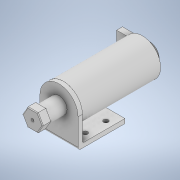
# Autodesk Inventor part: motor
Saved by Autodesk Inventor 2022 (Build 260153000, 153)
## iProperties
Created: 2022-07-16
Part Number: motor
Material: Типовые
Document SubType Name: Modeling
Designer: akapu
Density: 1 g/cm^3
Appearance: По умолчанию
Author: akapu
Autodesk Inventor part; units mm, degrees
ref_plane "YZ Plane" through (0, 0, 0) normal (1, 0, 0) x (0, 1, 0)
ref_plane "XZ Plane" through (0, 0, 0) normal (0, 1, 0) x (-1, 0, 0)
ref_plane "XY Plane" through (0, 0, 0) normal (0, 0, 1) x (1, 0, 0)
sketch "Эскиз1" plane through (0, 0, 0) normal (0, 1, 0) x (-1, 0, 0)
  line L0 (0, 0) -> (-26, 0)
  line L1 (0, -32) -> (-26, -32)
  line L2 (-26, -32) -> (0, -32)
  line L3 (0, -32) -> (0, 0)
  line L4 (0, 0) -> (-26, 0)
  line L5 (-26, 0) -> (-26, -32)
  constraints: 12 end point, 2 horizontal, 2 parallel, 1 perpendicular
extrude "Выдавливание1" add sketch "Эскиз1" along normal blind 3
sketch "Эскиз2" plane through (0, 3, 0) normal (0, 1, 0) x (1, 0, 0)
  line L0 (0, 0) -> (26, 0) projected
  line L1 (26, 0) -> (26, 33) projected
  line L2 (0, 0) -> (26, 0)
  line L3 (26, 0) -> (26, 3)
  line L4 (26, 3) -> (0, 3)
  line L5 (0, 3) -> (0, 0)
  dimension "d4" = 3
  constraints: 8 end point, 2 parallel, 1 horizontal, 1 perpendicular, 1 point on line
  measures "d4" distance of L3.end L2.end
extrude "Выдавливание2" add sketch "Эскиз2" along normal blind 30
sketch "Эскиз3" plane through (26, 3, -3) normal (0, 0, -1) x (-1, 0, 0)
  line L0 (0, 0) -> (26, 0) projected
  line L1 (13, 0) -> (13, 5)
  line L2 (13, 5) -> (13, 17.5)
  circle A0 centre (13, 17.5) radius 12.5
  point P0 (26, -3)
  dimension "d7" = 5
  dimension "d8" = 12.5
  constraints: 4 end point, 1 coincident, 1 midpoint, 1 point on line, 1 vertical, 1 vertical alignment, 2 other
  measures "d7" distance of L1.start L1.end
  measures "d8" distance of L1.end L2.end
extrude "Выдавливание3" add sketch "Эскиз3" along normal blind 61.8
sketch "Эскиз4" plane through (13, 20.5, -64.8) normal (0, 0, -1) x (-1, 0, 0)
  circle A0 centre (0, 0) radius 6.5
  circle A1 centre (0, 0) radius 12.5
  point P0 (13, -20.5)
  dimension "d11" = 13
  constraints: 2 centre point, 1 coincident
  measures "d11" diameter of A0
extrude "Выдавливание4" cut sketch "Эскиз4" against normal blind 8
sketch "Эскиз5" plane through (13, 20.5, -64.8) normal (0, 0, -1) x (-1, 0, 0)
  circle A0 centre (0, 0) radius 1
  circle A1 centre (0, 0) radius 6.5
  point P0 (13, -20.5)
  dimension "d14" = 2
  constraints: 2 centre point, 1 coincident
  measures "d14" diameter of A0
extrude "Выдавливание5" cut sketch "Эскиз5" against normal blind 3
sketch "Эскиз6" plane through (13, 20.5, -56.8) normal (0, 0, -1) x (-1, 0, 0)
  circle A0 centre (0, 0) radius 12.5 projected
  line L0 (-12.5, 0) -> (8.5, 0)
  line L1 (8.5, 0) -> (8.5, 7)
  line L2 (8.5, 7) -> (17.5, 7)
  line L3 (17.5, 7) -> (17.5, -7)
  line L4 (17.5, -7) -> (8.5, -7)
  line L5 (8.5, -7) -> (8.5, 0)
  point P0 (13, -20.5)
  dimension "d17" = 21
  dimension "d18" = 7
  dimension "d19" = 9
  dimension "d20" = 14
  constraints: 12 end point, 5 perpendicular, 1 horizontal, 1 horizontal alignment, 1 point on line, 1 other
  measures "d17" distance of L0.start L0.end
  measures "d18" distance of L0.end L1.end
  measures "d19" distance of L1.end L2.end
  measures "d20" distance of L2.end L3.end
extrude "Выдавливание6" add sketch "Эскиз6" along normal blind 4 contours A0 L4 L5 L1 L2 | A0 L2 L3 L4
sketch "Эскиз7" plane through (0, 0, 0) normal (0, 0, 1) x (1, 0, 0)
  circle A0 centre (13, 20.5) radius 1 projected
  circle A1 centre (13, 20.5) radius 5.5
  point P0 (0, 0)
  dimension "d23" = 11
  constraints: 1 centre point, 1 coincident
  measures "d23" diameter of A1
extrude "Выдавливание7" add sketch "Эскиз7" along normal blind 12 contours A0 | A1
sketch "Эскиз8" plane through (13, 20.5, 12) normal (0, 0, 1) x (1, 0, 0)
  line L0 (0, 0) -> (0, 6)
  circle A0 centre (0, 0) radius 1 projected
  line L1 (3.4641, 6) -> (6.9282, 0)
  line L2 (6.9282, 0) -> (3.4641, -6)
  line L3 (3.4641, -6) -> (-3.4641, -6)
  line L4 (-3.4641, -6) -> (-6.9282, 0)
  line L5 (-6.9282, 0) -> (-3.4641, 6)
  line L6 (-3.4641, 6) -> (3.4641, 6)
  point P0 (-13, -20.5)
  dimension "d26" = 6
  constraints: 14 end point, 1 coincident, 1 midpoint, 1 vertical, 13 other
  measures "d26" distance of L0.start L0.end
extrude "Выдавливание8" add sketch "Эскиз8" along normal blind 6
fillet "Сопряжение1" radius 0.5 12 edges at (7.8038, 23.5, 12) (13, 26.5, 12) (7.8038, 17.5, 12) (13, 14.5, 12) (18.1962, 17.5, 12) (18.1962, 23.5, 12) (13, 14.5, 18) (18.1962, 17.5, 18) (18.1962, 23.5, 18) (13, 26.5, 18) (7.8038, 23.5, 18) (7.8038, 17.5, 18)
sketch "Эскиз9" plane through (0, 0, 0) normal (0, -1, 0) x (1, 0, 0)
  line L0 (26, 0) -> (26, -33) projected
  line L1 (0, 0) -> (26, 0) projected
  line L2 (5, -10) -> (21, -10)
  line L3 (21, -10) -> (21, -24)
  line L4 (21, -24) -> (5, -24)
  line L5 (5, -24) -> (5, -10)
  circle A0 centre (5, -10) radius 1.6
  circle A1 centre (21, -10) radius 1.6
  circle A2 centre (21, -24) radius 1.6
  circle A3 centre (5, -24) radius 1.6
  dimension "d45" = 16
  dimension "d46" = 14
  dimension "d47" = 3.2
  dimension "d48" = 3.2
  dimension "d49" = 3.2
  dimension "d50" = 3.2
  constraints: 8 end point, 4 centre point, 4 coincident, 2 parallel, 1 horizontal, 1 perpendicular
  measures "d45" distance of L3.end L4.end
  measures "d46" distance of L2.end L3.end
  measures "d47" diameter of A0
  measures "d48" diameter of A1
  measures "d49" diameter of A2
  measures "d50" diameter of A3
extrude "Выдавливание9" cut sketch "Эскиз9" against normal blind 3 contours L5 A0 L2 | L2 A0 L5 | A1 L3 L2 | L2 L3 A1 | A3 L4 L5 | L5 L4 A3 | A2 L4 L3 | L3 L4 A2
fillet "Сопряжение2" radius 2 1 edges at (13, 0, 0)
fillet "Сопряжение3" radius 1 1 edges at (13, 3, -3)
fillet "Сопряжение4" radius 13 2 edges at (0, 33, -1.5) (26, 33, -1.5)
